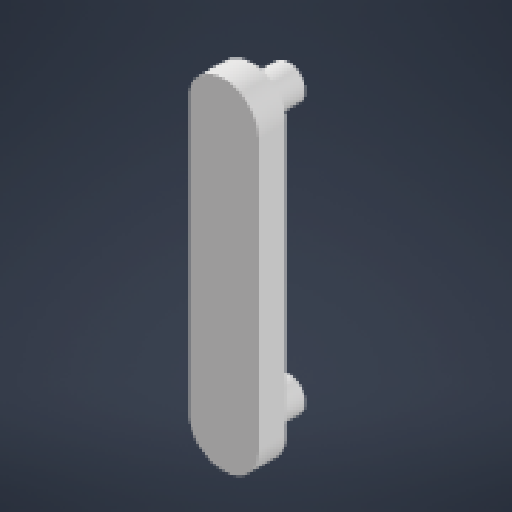
# Autodesk Inventor part: Колено
Saved by Autodesk Inventor 2026 (Build 300175000, 175)
## iProperties
Created: 2026-04-19
Part Number: Колено
Material: Типовые
Document SubType Name: Modeling
Designer: Artem Sannikov
Density: 1 g/cm^3
Appearance: По умолчанию
Author: Artem Sannikov
Autodesk Inventor part; units mm, degrees
ref_plane "YZ Plane" through (0, 0, 0) normal (1, 0, 0) x (0, 1, 0)
ref_plane "XZ Plane" through (0, 0, 0) normal (0, 1, 0) x (-1, 0, 0)
ref_plane "XY Plane" through (0, 0, 0) normal (0, 0, 1) x (1, 0, 0)
sketch "Эскиз1" plane through (0, 0, 0) normal (0, 0, 1) x (1, 0, 0)
  circle A0 centre (0, -10) radius 9 projected
  circle A1 centre (0, -10) radius 14.5552
  point P0 (0, 0)
  constraints: 1 centre point, 1 coincident
extrude "Выдавливание1" add sketch "Эскиз1" along normal blind 31.5 contours A0 | A1
sketch "Эскиз2" plane through (0, -10, 31.5) normal (0, 0, 1) x (1, 0, 0)
  line L0 (0, 0) -> (0, 230) construction
  line L1 (30, 0) -> (30, 230)
  line L2 (-30, 230) -> (-30, 0)
  arc A0 (-30, 0) -> (30, 0) centre (0, 0) ccw
  arc A1 (30, 230) -> (-30, 230) centre (0, 230) ccw
  circle A2 centre (0, 0) radius 14.5552 projected
  point P0 (0, 10)
  point P1 (0, 115)
  dimension "d4" = 230
  dimension "d5" = 30
  constraints: 8 end point, 4 point on circle, 4 tangent, 2 centre point, 1 coincident, 1 midpoint, 1 parallel, 1 vertical
  measures "d4" distance of L0.end L0.start
  measures "d5" radius of A0
extrude "Выдавливание2" add sketch "Эскиз2" along normal blind 24 contours A0 L2 A1 L1 | A2
sketch "Эскиз3" plane through (0, -10, 31.5) normal (0, 0, -1) x (-1, 0, 0)
  circle A0 centre (0, 230) radius 14.555
  arc A1 (30, 230) -> (-30, 230) centre (0, 230) ccw projected
  point P0 (0, 10)
  dimension "d6" = 29.11
  constraints: 1 centre point, 1 coincident
  measures "d6" diameter of A0
extrude "Выдавливание3" add sketch "Эскиз3" along normal up to surface (31.5 mm away)
sketch "Эскиз4" plane through (0, -10, 55.5) normal (0, 0, 1) x (1, 0, 0)
  arc A0 (30, 230) -> (-30, 230) centre (0, 230) ccw projected
  line L0 (-30, 230) -> (-30, 0) projected
  arc A1 (-30, 0) -> (30, 0) centre (0, 0) ccw projected
  line L1 (30, 0) -> (30, 230) projected
  circle A2 centre (0, 115) radius 10
  point P0 (0, 10)
  dimension "d9" = 20
  constraints: 1 centre point
  measures "d9" diameter of A2
extrude "Выдавливание4" cut sketch "Эскиз4" against normal blind 5 contours A2
